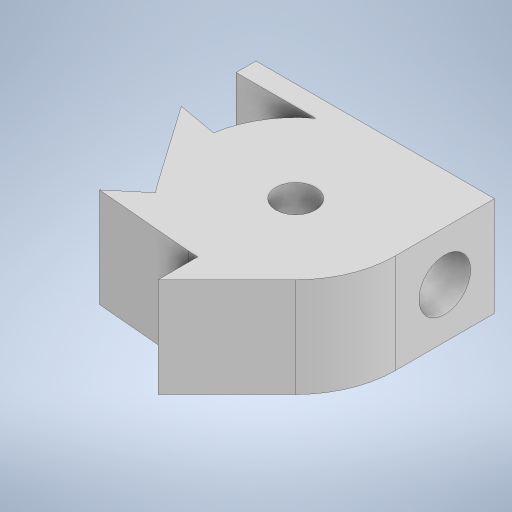
# Autodesk Inventor part: exp_latch_rod_rev0
Saved by Autodesk Inventor 2024 (Build 280153000, 153)
## iProperties
Created: 2024-04-11
Part Number: exp_latch_rod_rev0
Material: 一般
Document SubType Name: Modeling
Designer: Akio
Density: 1 g/cm^3
Appearance: 既定
Author: Akio
Autodesk Inventor part; units mm, degrees
ref_plane "YZ Plane" through (0, 0, 0) normal (1, 0, 0) x (0, 1, 0)
ref_plane "XZ Plane" through (0, 0, 0) normal (0, 1, 0) x (-1, 0, 0)
ref_plane "XY Plane" through (0, 0, 0) normal (0, 0, 1) x (1, 0, 0)
sketch "スケッチ1" plane through (0, 0, 0) normal (0, 1, 0) x (-1, 0, 0)
  arc A0 (0, -5) -> (-5, 0) centre (0, 0) ccw
  line L0 (0, -5) -> (-5, -5)
  line L1 (0, -5) -> (5, -5) construction
  line L2 (-5, -5) -> (-5, 0)
  dimension "d1" = 5
  dimension "d2" = 5
  dimension "d3" = 180
  dimension "d4" = 5
  constraints: 6 end point, 3 point on circle, 2 horizontal, 1 centre point, 1 coincident, 1 collinear
  measures "d1" distance of L2.end point (0, 0)
  measures "d2" distance of L0.start L0.end
  measures "d3" angle of L0 L1
  measures "d4" distance of L0.end L2.end
extrude "押し出し1" add sketch "スケッチ1" along normal blind 5
sketch "スケッチ2" plane through (0, 5, 0) normal (0, 1, 0) x (1, 0, 0)
  arc A0 (0, 5) -> (5, 0) centre (0, 0) ccw projected
  line L0 (0.0716, -4.9995) -> (0.0716, -6.9995)
  line L1 (0.0716, -6.9995) -> (3.5355, -3.5355)
  line L2 (0.0716, -6.9995) -> (4.9704, -6.9995) construction
  line L3 (0.0716, -4.9995) -> (3.5355, -3.5355)
  dimension "d7" = 2
  dimension "d8" = 45
  constraints: 8 end point, 3 point on circle, 1 equal length, 1 horizontal, 1 tangent, 1 vertical
  measures "d7" distance of L0.start L0.end
  measures "d8" angle of L2 L1
extrude "押し出し2" add sketch "スケッチ2" against normal blind 5 contours A0 L1 L0
pattern_circular "円形状パターン1" count 3 over 100 about axis through (0, 0, 0) along (0, -1, 0) of "押し出し2"
sketch "スケッチ3" plane through (0, 5, 0) normal (0, 1, 0) x (1, 0, 0)
  point P0 (0, 0)
  point P1 (0, 0)
  constraints: 1 coincident
hole "穴1" at (0, 5, 0) direction (0, -1, 0) diameter 2 end through all
sketch "スケッチ4" plane through (5, 0, 0) normal (1, 0, 0) x (0, 0, -1)
  line L0 (0, 5) -> (5, 5) projected
  line L1 (5, 0) -> (5, 5) projected
  point P0 (0, 0)
  point P1 (2.5, 2.5)
  dimension "d28" = 2.5
  dimension "d29" = 2.5
  measures "d28" distance from line of L0 point (2.5, 2.5)
  measures "d29" distance from line of L1 point (2.5, 2.5)
hole "穴2" at (5, 2.5, -2.5) direction (-1, 0, 0) diameter 2.6 depth 5
sketch "スケッチ5" plane through (0, 5, 0) normal (0, 1, 0) x (1, 0, 0)
  point P0 (0, 0)
sketch "スケッチ7" plane through (0, 5, 0) normal (0, 1, 0) x (1, 0, 0)
  arc A0 (0, 5) -> (-4.936, 0.7977) centre (0, 0) ccw projected
  line L0 (0, 5) -> (-7, 5)
  line L1 (-7, 5) -> (-7, 4)
  line L2 (-7, 4) -> (-3, 4)
  line L3 (-3, 4) -> (0, 5)
  dimension "d35" = 7
  dimension "d36" = 1
  constraints: 8 end point, 1 horizontal, 1 perpendicular, 1 point on circle, 1 tangent, 1 vertical
  measures "d35" distance of L0.start L0.end
  measures "d36" distance of L0.end L1.end
extrude "押し出し4" add sketch "スケッチ7" against normal blind 5 contours A0 L2 L1 L0
